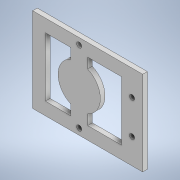
# Autodesk Inventor part: BASE
Saved by Autodesk Inventor 2022 (Build 260153000, 153)
## iProperties
Created: 2022-11-02
Part Number: BASE
Material: Genérico
Document SubType Name: Modeling
Designer: Usuario
Density: 1 g/cm^3
Appearance: Valor por defecto
Author: Usuario
Autodesk Inventor part; units mm, degrees
ref_plane "YZ Plane" through (0, 0, 0) normal (1, 0, 0) x (0, 1, 0)
ref_plane "XZ Plane" through (0, 0, 0) normal (0, 1, 0) x (-1, 0, 0)
ref_plane "XY Plane" through (0, 0, 0) normal (0, 0, 1) x (1, 0, 0)
sketch "Boceto1" plane through (0, 0, 0) normal (0, 0, 1) x (1, 0, 0)
  line L0 (-65, -50) -> (65, -50)
  line L1 (65, -50) -> (65, 50)
  line L2 (65, 50) -> (-65, 50)
  line L3 (-65, 50) -> (-65, -50)
  line L4 (-65, -50) -> (65, 50) construction
  line L5 (65, -50) -> (-65, 50) construction
  line L6 (-50, -35) -> (50, -35)
  line L7 (50, -35) -> (50, 35)
  line L8 (50, 35) -> (-50, 35)
  line L9 (-50, 35) -> (-50, -35)
  line L10 (-50, -35) -> (50, 35) construction
  line L11 (50, -35) -> (-50, 35) construction
  point P0 (0, 0)
  dimension "d0" = 130
  dimension "d1" = 100
  dimension "d2" = 100
  dimension "d3" = 70
  constraints: 24 end point, 4 midpoint, 4 parallel, 2 horizontal, 2 perpendicular
  measures "d0" distance of L2.end L1.end
  measures "d1" distance of L1.end L0.end
  measures "d2" distance of L8.end L7.end
  measures "d3" distance of L7.end L6.end
extrude "Extrusión1" add sketch "Boceto1" along normal blind 5.5
sketch "Boceto2" plane through (0, 0, 0) normal (0, 0, 1) x (1, 0, 0)
  line L0 (0, 0) -> (-20, 0)
  line L1 (-20, 0) -> (-20, 35)
  line L2 (-50, 35) -> (50, 35) projected
  line L3 (-20, 0) -> (0, 0)
  line L4 (0, 0) -> (0, 35)
  line L5 (0, 35) -> (-20, 35)
  line L6 (-20, 35) -> (-20, 0)
  line L7 (50, -35) -> (-50, -35) projected
  line L8 (-20, 0) -> (0, 0)
  line L9 (0, 0) -> (0, -35)
  line L10 (0, -35) -> (-20, -35)
  line L11 (-20, -35) -> (-20, 0)
  line L12 (50, 35) -> (40, 35)
  line L13 (40, 35) -> (40, -35)
  line L14 (50, 35) -> (50, -35) projected
  line L15 (50, -35) -> (50, 35)
  line L16 (50, -35) -> (40, -35)
  dimension "d6" = 20
  dimension "d7" = 10
  constraints: 28 end point, 4 horizontal, 4 parallel, 4 perpendicular, 3 point on line, 2 midpoint, 1 vertical
  measures "d6" distance of L0.start L0.end
  measures "d7" distance of L2.end L12.end
extrude "Extrusión9" add sketch "Boceto2" along normal blind 5.5 contours L9 L7 L11 L0 | L0 L1 L2 L4 | L2 L14 L7 L13
sketch "Boceto8" plane through (0, 0, 5.5) normal (0, 0, 1) x (1, 0, 0)
  line L0 (0, 0) -> (-20, 0)
  line L1 (-20, 35) -> (-20, -35) projected
  line L2 (-10, 0) -> (-10, 50)
  line L3 (65, 50) -> (-65, 50) projected
  line L4 (0, 35) -> (-10, 35)
  line L5 (-10, 35) -> (-10, 50)
  line L6 (-10, 50) -> (-10, 42.5)
  line L7 (-10, 0) -> (65, 0)
  line L8 (65, -50) -> (65, 50) projected
  line L9 (40, 35) -> (40, -35) projected
  line L10 (40, 0) -> (65, 0)
  line L11 (52.5, 0) -> (52.5, 20)
  circle A0 centre (-10, 42.5) radius 3
  circle A1 centre (52.5, 20) radius 3
  circle A2 centre (-10, -42.5) radius 3
  circle A3 centre (52.5, -20) radius 3
  dimension "d32" = 20
  dimension "d33" = 6
  dimension "d34" = 6
  constraints: 16 end point, 6 midpoint, 4 centre point, 3 perpendicular, 2 coincident, 2 point on line, 2 symmetric about line, 1 collinear, 1 vertical, 2 other
  measures "d32" distance of L11.start L11.end
  measures "d33" diameter of A0
  measures "d34" diameter of A1
extrude "Extrusión10" cut sketch "Boceto8" against normal blind 5.5 contours A1 | A0 L2 | L2 A0 | A2 | A3
sketch "Boceto9" plane through (0, 0, 5.5) normal (0, 0, 1) x (1, 0, 0)
  line L0 (-20, 35) -> (-20, -35) projected
  line L1 (-20, 0) -> (0, 0)
  circle A0 centre (-10, 0) radius 25
  dimension "d40" = 50
  constraints: 2 end point, 2 midpoint, 1 centre point, 1 horizontal
  measures "d40" diameter of A0
extrude "Extrusión12" add sketch "Boceto9" against normal blind 5.5
